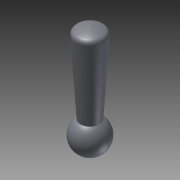
# Autodesk Inventor part: 01
Saved by Autodesk Inventor 2012 (Build 160160000, 160)
## iProperties
Created: 2014-01-27
Part Number: 01
Material: Default
Document SubType Name: Modeling
Designer: Michał
Density: 1 g/cm^3
Author: Michał
Autodesk Inventor part; units mm, degrees
ref_plane "YZ Plane" through (0, 0, 0) normal (1, 0, 0) x (0, 1, 0)
ref_plane "XZ Plane" through (0, 0, 0) normal (0, 1, 0) x (-1, 0, 0)
ref_plane "XY Plane" through (0, 0, 0) normal (0, 0, 1) x (1, 0, 0)
sketch "Sketch2" plane through (0, 0, 0) normal (1, 0, 0) x (0, 1, 0)
  arc A0 (0, -3.5) -> (2, 2.8723) centre (0, 0) ccw
  line L0 (2, 2.8723) -> (3, 18.8723)
  arc A1 (3, 18.8723) -> (0, 19.8285) centre (-0.5142, 13.0309) ccw
  line L1 (0, -3.5) -> (0, 19.8285)
  dimension "d0" = 3.5
  dimension "d2" = 3
  dimension "d3" = 16
  dimension "d6" = 2
  constraints: 5 point on circle, 4 end point, 2 centre point, 1 coincident
  measures "d0" radius of A0
  measures "d2" horizontal distance of L0.end point (0, 0)
  measures "d3" vertical distance of L0.start L0.end
  measures "d6" horizontal distance of point (0, 0) L0.start
revolve "Revolution1" add sketch "Sketch2" angle 360 about axis through (0, 0, -3.5) along (0, 0, 1)
fillet "Fillet1" radius 1 1 edges at (0, -3, 18.8723)
body "Solid1"
